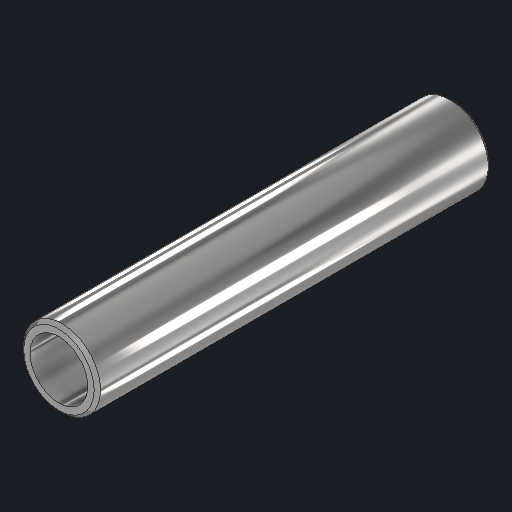
# Autodesk Inventor part: motor_driveshaft
Saved by Autodesk Inventor 2027.1 (Build 311270010, 270A)
## iProperties
Created: 2026-10-08
Part Number: motor_driveshaft
Material: Steel
Document SubType Name: Modeling
Designer: luca
Density: 7.85 g/cm^3
Appearance: Stahl - poliert
Author: luca
Autodesk Inventor part; units mm, degrees
ref_plane "YZ Plane" through (0, 0, 0) normal (1, 0, 0) x (0, 1, 0)
ref_plane "XZ Plane" through (0, 0, 0) normal (0, 1, 0) x (-1, 0, 0)
ref_plane "XY Plane" through (0, 0, 0) normal (0, 0, 1) x (1, 0, 0)
sketch "Skizze1" plane through (0, 0, 0) normal (0, 1, 0) x (-1, 0, 0)
  circle A0 centre (0, 0) radius 6
  circle A1 centre (0, 0) radius 4.5
  dimension "d0" = 12
  dimension "d6" = 9
  constraints: 2 centre point, 2 coincident
  measures "d0" diameter of A0
  measures "d6" diameter of A1
extrude "Extrusion1" add sketch "Skizze1" along normal blind 61.5
chamfer "Fasen1" distance 0.5 angle 45 2 edges at (6, 61.5, 0) (6, 0, 0)
